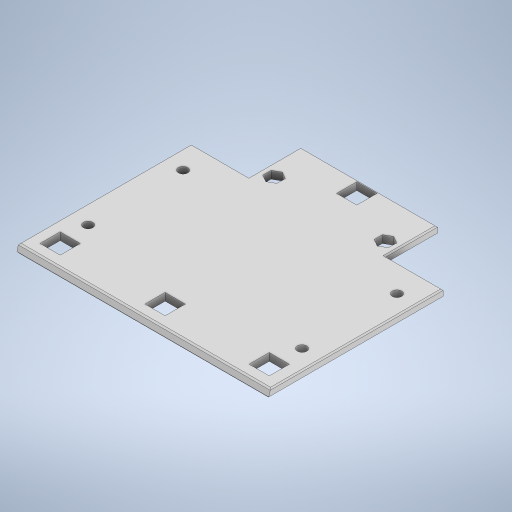
# Autodesk Inventor part: Plech pro celý spodek
Saved by Autodesk Inventor 2024 (Build 280153000, 153)
## iProperties
Created: 2023-09-06
Part Number: Plech pro celý spodek
Material: Všeobecné
Document SubType Name: Modeling
Designer: Simak
Density: 1 g/cm^3
Appearance: Výchozí
Author: Simak
Autodesk Inventor part; units mm, degrees
ref_plane "YZ Plane" through (0, 0, 0) normal (1, 0, 0) x (0, 1, 0)
ref_plane "XZ Plane" through (0, 0, 0) normal (0, 1, 0) x (-1, 0, 0)
ref_plane "XY Plane" through (0, 0, 0) normal (0, 0, 1) x (1, 0, 0)
sketch "Náčrt1" plane through (0, 0, 0) normal (0, 1, 0) x (-1, 0, 0)
  line L0 (49.75, -19.25) -> (49.75, 49.75)
  line L1 (49.75, 49.75) -> (-49.75, 49.75)
  line L2 (-49.75, 49.75) -> (-49.75, -19.25)
  line L3 (-49.75, -19.25) -> (-27, -19.25)
  line L4 (-27, -19.25) -> (-27, -49.75)
  line L5 (-27, -49.75) -> (27, -49.75)
  line L6 (27, -49.75) -> (27, -19.25)
  line L7 (27, -19.25) -> (49.75, -19.25)
  point P0 (0, 0)
  dimension "d0" = 30.5
  dimension "d1" = 99.5
  dimension "d2" = 22.75
  dimension "d3" = 99.5
  dimension "d4" = 54
  dimension "d5" = 49.75
  dimension "d6" = 49.75
  constraints: 16 end point, 6 perpendicular, 2 vertical, 1 parallel
  measures "d0" distance of L3.end L4.end
  measures "d1" distance of L0.end L1.end
  measures "d2" distance of L2.end L3.end
  measures "d3" distance between parallel lines of L1 L5
  measures "d4" distance of L4.end L5.end
  measures "d5" horizontal distance of L1.end point (0, 0)
  measures "d6" distance from line of point (0, 0) L1
extrude "Vysunutí1" add sketch "Náčrt1" along normal blind 3
sketch "Náčrt2" plane through (27, 0, -19.25) normal (1, 0, 0) x (0, 0, -1)
  line L0 (30.5, 3) -> (0, 3) projected
  line L1 (0, 3) -> (0, 11)
  line L2 (0, 11) -> (9.875, 11)
  line L3 (9.875, 11) -> (9.875, 7.646)
  arc A0 (9.875, 7.646) -> (20.625, 7.646) centre (15.25, 10.5828) ccw
  line L4 (20.625, 7.646) -> (20.625, 11)
  line L5 (20.625, 11) -> (30.5, 11)
  line L6 (30.5, 11) -> (30.5, 3)
  line L7 (0, 0) -> (30.5, 0) projected
  point P0 (-19.25, 0)
  dimension "d9" = 6.125
  dimension "d10" = 11
  dimension "d11" = 9.875
  dimension "d12" = 3.354
  constraints: 12 end point, 3 perpendicular, 2 equal length, 2 point on circle, 2 point on line, 1 centre point, 1 parallel, 1 vertical
  measures "d9" radius of A0
  measures "d10" distance between parallel lines of L5 L7
  measures "d11" distance of L4.end L5.end
  measures "d12" distance of L4.start L4.end
extrude "Vysunutí2" add sketch "Náčrt2" against normal up to surface (54 mm away)
sketch "Náčrt3" plane through (27, 3, -19.25) normal (0, 0, 1) x (1, 0, 0)
  line L0 (0, 8) -> (-54, 8) projected
  line L1 (-39, 8) -> (-39, 0)
  line L2 (-15, 8) -> (-15, 0)
  line L3 (-76.75, 0) -> (22.75, 0) projected
  line L4 (0, 8) -> (0, 0) projected
  line L5 (-54, 8) -> (-54, 0) projected
  line L6 (-15, 4) -> (0, 4)
  line L7 (-39, 4) -> (-54, 4)
  point P0 (-27, -3)
  dimension "d24" = 24
  constraints: 8 end point, 4 midpoint, 4 point on line, 2 vertical, 1 collinear
  measures "d24" distance between parallel lines of L1 L2
extrude "Vysunutí3" cut sketch "Náčrt3" against normal up to surface (20.625 mm away) contours L2 L3 L1 L0
sketch "Náčrt4" plane through (-27, 3, -19.25) normal (0, 0, 1) x (1, 0, 0)
  line L0 (0, 1.4578) -> (15, 1.4578) projected
  line L1 (39, 1.4578) -> (54, 1.4578) projected
  line L2 (10, 1.4578) -> (10, 8)
  line L3 (54, 8) -> (0, 8) projected
  line L4 (0, 8) -> (0, 0) projected
  line L5 (44, 8) -> (44, 1.4578)
  line L6 (54, 8) -> (54, 0) projected
  line L7 (15, 0) -> (15, 8) projected
  line L8 (39, 8) -> (39, 0) projected
  point P0 (27, -3)
  dimension "d20" = 10
  dimension "d21" = 10
  constraints: 4 end point, 4 point on line, 2 vertical
  measures "d20" distance between parallel lines of L4 L2
  measures "d21" distance between parallel lines of L6 L5
extrude "Vysunutí4" cut sketch "Náčrt4" against normal up to next contours L2 L3 L7 L0 | L8 L3 L5 L1
sketch "Náčrt5" plane through (-27, 3, -19.25) normal (0, 0, 1) x (1, 0, 0)
  line L0 (10, 1.4578) -> (10, 0)
  line L1 (15, 0) -> (0, 0) projected
  line L2 (44, 1.4578) -> (44, 0)
  line L3 (54, 0) -> (39, 0) projected
  line L4 (15, 1.4578) -> (10, 1.4578) projected
  line L5 (15, 0) -> (15, 1.4578) projected
  line L6 (-22.75, 0) -> (76.75, 0) projected
  line L7 (39, 1.4578) -> (39, 0) projected
  line L8 (44, 1.4578) -> (39, 1.4578) projected
  point P0 (27, -3)
  constraints: 4 end point, 2 coincident, 2 point on line, 1 parallel, 1 vertical
extrude "Vysunutí5" cut sketch "Náčrt5" against normal blind 6.875
sketch "Náčrt6" plane through (27, 7.646, -39.875) normal (0, 0, 1) x (1, 0, 0)
  line L0 (0, 3.354) -> (-54, 3.354) projected
  line L1 (-37, 3.354) -> (-37, -3.646)
  line L2 (-37, -3.646) -> (-17, -3.646)
  line L3 (-17, -3.646) -> (-17, 3.354)
  line L4 (-76.75, -4.646) -> (22.75, -4.646) projected
  line L5 (0, 3.354) -> (0, 0) projected
  line L6 (-17, -0.146) -> (0, -0.146) construction
  line L7 (-37, -0.146) -> (-54, -0.146) construction
  line L8 (-54, -7.646) -> (-54, 3.354) projected
  point P0 (-27, -7.646)
  dimension "d27" = 1
  dimension "d35" = 20
  constraints: 10 end point, 4 point on line, 2 horizontal, 2 midpoint, 2 perpendicular, 1 collinear, 1 vertical
  measures "d27" distance between parallel lines of L4 L2
  measures "d35" distance of L1.end L2.end
extrude "Vysunutí6" cut sketch "Náčrt6" against normal up to next
sketch "Náčrt7" plane through (-27, 11, -19.25) normal (0, 1, 0) x (1, 0, 0)
  circle A0 centre (5, 4.9375) radius 1.85
  circle A1 centre (5, 25.5625) radius 1.85
  circle A2 centre (49, 25.5625) radius 1.85
  circle A3 centre (49, 4.9375) radius 1.85
  line L0 (76.75, 0) -> (54, 0) projected
  line L1 (49, 4.9375) -> (54, 0) construction
  line L2 (54, 0) -> (44, 0) projected
  line L3 (44, 0) -> (49, 4.9375) construction
  line L4 (54, 9.875) -> (49, 4.9375) construction
  line L5 (10, 0) -> (10, 6.875) projected
  line L6 (5, 4.9375) -> (10, 0) construction
  line L7 (0, 30.5) -> (0, 0) projected
  line L8 (0, 0) -> (5, 4.9375) construction
  line L9 (5, 4.9375) -> (0, 9.875) construction
  line L10 (0, 20.625) -> (5, 25.5625) construction
  line L11 (5, 25.5625) -> (0, 30.5) construction
  line L12 (54, 0) -> (54, 30.5) projected
  line L13 (54, 20.625) -> (49, 25.5625) construction
  line L14 (49, 25.5625) -> (54, 30.5) construction
  point P0 (27, -19.25)
  dimension "d6" = 49.75
  dimension "d36" = 3.7
  constraints: 20 end point, 12 equal length, 4 centre point, 3 equal radius, 1 coincident
  measures "d36" diameter of A1
extrude "Vysunutí7" cut sketch "Náčrt7" against normal through all
sketch "Náčrt27" plane through (0, 0, 0) normal (0, -1, 0) x (1, 0, 0)
  circle A0 centre (22, -44.8125) radius 1.85 projected
  line L0 (19.175, -43.1815) -> (22, -41.5505)
  line L1 (22, -41.5505) -> (24.825, -43.1815)
  line L2 (24.825, -43.1815) -> (24.825, -46.4435)
  line L3 (24.825, -46.4435) -> (22, -48.0745)
  line L4 (22, -48.0745) -> (19.175, -46.4435)
  line L5 (19.175, -46.4435) -> (19.175, -43.1815)
  line L6 (19.175, -25.8185) -> (19.175, -22.5565)
  line L7 (19.175, -22.5565) -> (22, -20.9255)
  line L8 (22, -20.9255) -> (24.825, -22.5565)
  line L9 (24.825, -22.5565) -> (24.825, -25.8185)
  line L10 (24.825, -25.8185) -> (22, -27.4495)
  line L11 (22, -27.4495) -> (19.175, -25.8185)
  circle A1 centre (-22, -24.1875) radius 1.85 projected
  line L12 (-19.175, -25.8185) -> (-22, -27.4495)
  line L13 (-22, -27.4495) -> (-24.825, -25.8185)
  line L14 (-24.825, -25.8185) -> (-24.825, -22.5565)
  line L15 (-24.825, -22.5565) -> (-22, -20.9255)
  line L16 (-22, -20.9255) -> (-19.175, -22.5565)
  line L17 (-19.175, -22.5565) -> (-19.175, -25.8185)
  circle A2 centre (-22, -44.8125) radius 1.85 projected
  line L18 (-19.175, -46.4435) -> (-22, -48.0745)
  line L19 (-22, -48.0745) -> (-24.825, -46.4435)
  line L20 (-24.825, -46.4435) -> (-24.825, -43.1815)
  line L21 (-24.825, -43.1815) -> (-22, -41.5505)
  line L22 (-22, -41.5505) -> (-19.175, -43.1815)
  line L23 (-19.175, -43.1815) -> (-19.175, -46.4435)
  point P0 (0, 0)
  point P1 (22, -24.1875)
  dimension "d179" = 5.65
  constraints: 48 end point, 4 vertical, 3 coincident, 3 equal length, 1 horizontal alignment, 1 vertical alignment, 52 other
  measures "d179" distance between parallel lines of L2 L5
extrude "Vysunutí30" cut sketch "Náčrt27" against normal blind 7 contours A0 | L0 L1 L2 L3 L4 L5 | L6 L7 L8 L9 L10 L11 | A1 | L12 L13 L14 L15 L16 L17 | A2 | L18 L19 L20 L21 L22 L23
chamfer "Zkosení2" distance 1 angle 45 4 edges at (20.15, 7, -44.8125) (20.15, 7, -24.1875) (-23.85, 7, -24.1875) (-23.85, 7, -44.8125)
sketch "Náčrt28" plane through (0, 3, 0) normal (0, 1, 0) x (1, 0, 0)
  circle A0 centre (-42.25, 8.5) radius 1.85
  circle A1 centre (42.25, 8.5) radius 1.85
  circle A2 centre (42.25, -29) radius 1.85
  circle A3 centre (-42.25, -29) radius 1.85
  line L0 (-42.25, 8.5) -> (-49.75, 8.5) construction
  line L1 (-49.75, 19.25) -> (-49.75, -49.75) projected
  line L2 (42.25, 8.5) -> (49.75, 8.5) construction
  line L3 (49.75, -49.75) -> (49.75, 19.25) projected
  line L4 (-49.75, -49.75) -> (49.75, -49.75) projected
  point P0 (0, 0)
  dimension "d185" = 3.7
  dimension "d186" = 84.5
  dimension "d187" = 37.5
  dimension "d195" = 20.75
  constraints: 4 centre point, 4 end point, 3 equal radius, 3 point on line, 2 horizontal alignment, 2 vertical alignment, 1 collinear, 1 horizontal
  measures "d185" diameter of A0
  measures "d186" distance of L2.start L0.start
  measures "d187" distance of A3.centre L0.start
  measures "d195" distance from line of L4 A3.centre
sketch "Náčrt29" plane through (49.75, 0, 49.75) normal (1, 0, 0) x (0, 0, -1)
  line L0 (0, 0) -> (69, 0) projected
  line L1 (0, 0) -> (6.6987, 25)
  line L2 (6.6987, 25) -> (9.8046, 25)
  line L3 (9.8046, 25) -> (3.9097, 3)
  line L4 (0, 3) -> (69, 3) projected
  line L5 (0, 0) -> (0, 3) projected
  point P0 (49.75, 0)
  point P1 (0.8038, 3)
  dimension "d188" = 75
  dimension "d189" = 25
  dimension "d190" = 3
  constraints: 6 end point, 1 horizontal, 1 parallel, 1 point on line
  measures "d188" angle of L0 L1
  measures "d189" distance between parallel lines of L0 L2
  measures "d190" distance between parallel lines of L1 L3
extrude "Vysunutí31" add sketch "Náčrt29" against normal up to surface (99.5 mm away) contours L1 L2 L3 L4
extrude "Vysunutí32" cut sketch "Náčrt29" against normal through all contours L5 L4 L1
extrude "Vysunutí33" cut sketch "Náčrt28" against normal up to next
sketch "Náčrt31" plane through (0, 3, 0) normal (0, 1, 0) x (1, 0, 0)
  line L0 (37.136, -36.833) -> (45.136, -36.833)
  line L1 (45.136, -36.833) -> (45.136, -44.833)
  line L2 (45.136, -44.833) -> (37.136, -44.833)
  line L3 (37.136, -44.833) -> (37.136, -36.833)
  line L4 (-4, -36.833) -> (4, -36.833)
  line L5 (4, -36.833) -> (4, -44.833)
  line L6 (4, -44.833) -> (-4, -44.833)
  line L7 (-4, -44.833) -> (-4, -36.833)
  line L8 (-45.463, -36.833) -> (-37.463, -36.833)
  line L9 (-37.463, -36.833) -> (-37.463, -44.833)
  line L10 (-37.463, -44.833) -> (-45.463, -44.833)
  line L11 (-45.463, -44.833) -> (-45.463, -36.833)
  line L12 (49.75, -45.8403) -> (49.75, 19.25) projected
  line L13 (-49.75, 19.25) -> (-49.75, -45.8403) projected
  line L14 (-49.75, -49.75) -> (49.75, -49.75) projected
  line L15 (4, 38.875) -> (-4, 38.875)
  line L16 (-4, 38.875) -> (-4, 30.875)
  line L17 (-4, 30.875) -> (4, 30.875)
  line L18 (4, 30.875) -> (4, 38.875)
  line L19 (27, 39.875) -> (10, 39.875) projected
  line L20 (4, 34.875) -> (27, 34.875) construction
  line L21 (-4, 34.875) -> (-27, 34.875) construction
  line L22 (-27, 49.75) -> (-27, 19.25) projected
  line L23 (27, 19.25) -> (27, 49.75) projected
  point P0 (0, 0)
  point P1 (0, -36.833)
  dimension "d198" = 8
  dimension "d199" = 4.614
  dimension "d200" = 4.287
  dimension "d201" = 4.917
  dimension "d334" = 1
  constraints: 36 end point, 8 equal length, 8 parallel, 6 horizontal, 4 perpendicular, 3 midpoint, 3 point on line, 2 horizontal alignment, 1 vertical alignment
  measures "d198" distance between parallel lines of L2 L0
  measures "d199" distance between parallel lines of L12 L1
  measures "d200" distance between parallel lines of L13 L11
  measures "d201" distance from line of L14 L5.end
  measures "d334" distance between parallel lines of L15 L19
extrude "Vysunutí34" cut sketch "Náčrt31" against normal up to next
sketch "Náčrt32" plane through (-27, 0, -19.25) normal (0, 0, -1) x (-1, 0, 0)
  line L0 (0, 0) -> (22.75, 0) projected
  line L1 (22.75, 0) -> (20.25, 0)
  line L2 (20.25, 0) -> (20.25, 25)
  line L3 (20.25, 25) -> (22.75, 25)
  line L4 (22.75, 25) -> (22.75, 0)
  line L5 (-76.75, 0) -> (-74.25, 0)
  line L6 (-74.25, 0) -> (-74.25, 25)
  line L7 (-74.25, 25) -> (-76.75, 25)
  line L8 (-76.75, 25) -> (-76.75, 0)
  line L9 (-76.75, 25) -> (22.75, 25) projected
  point P0 (-27, 0)
  point P1 (20.25, 0)
  dimension "d204" = 2.5
  constraints: 16 end point, 4 parallel, 2 horizontal, 2 perpendicular, 1 collinear, 1 point on line
  measures "d204" distance between parallel lines of L2 L4
extrude "Vysunutí35" add sketch "Náčrt32" against normal up to next
sketch "Náčrt34" plane through (0, 3, 0) normal (0, 1, 0) x (1, 0, 0)
  circle A0 centre (42.25, -29) radius 1.85 projected
  circle A1 centre (42.25, 8.5) radius 1.85 projected
  circle A2 centre (-42.25, 8.5) radius 1.85 projected
  circle A3 centre (-42.25, -29) radius 1.85 projected
  circle A4 centre (42.25, -29) radius 3.5
  circle A5 centre (42.25, 8.5) radius 3.5
  circle A6 centre (-42.25, 8.5) radius 3.5
  circle A7 centre (-42.25, -29) radius 3.5
  point P0 (0, 0)
  dimension "d214" = 7
  constraints: 4 centre point, 4 coincident, 3 equal radius
  measures "d214" diameter of A4
extrude "Vysunutí37" add sketch "Náčrt34" along normal blind 4
sketch "Náčrt35" plane through (0, 0, 0) normal (0, -1, 0) x (1, 0, 0)
  line L0 (19.175, -25.8185) -> (19.175, -22.5565) projected
  circle A0 centre (42.25, -8.5) radius 1.85 projected
  line L1 (39.425, -10.131) -> (39.425, -6.869)
  line L2 (39.425, -6.869) -> (42.25, -5.238)
  line L3 (42.25, -5.238) -> (45.075, -6.869)
  line L4 (45.075, -6.869) -> (45.075, -10.131)
  line L5 (45.075, -10.131) -> (42.25, -11.762)
  line L6 (42.25, -11.762) -> (39.425, -10.131)
  circle A1 centre (42.25, 29) radius 1.85 projected
  line L7 (39.425, 27.369) -> (39.425, 30.631)
  line L8 (39.425, 30.631) -> (42.25, 32.262)
  line L9 (42.25, 32.262) -> (45.075, 30.631)
  line L10 (45.075, 30.631) -> (45.075, 27.369)
  line L11 (45.075, 27.369) -> (42.25, 25.738)
  line L12 (42.25, 25.738) -> (39.425, 27.369)
  circle A2 centre (-42.25, 29) radius 1.85 projected
  line L13 (-45.075, 27.369) -> (-45.075, 30.631)
  line L14 (-45.075, 30.631) -> (-42.25, 32.262)
  line L15 (-42.25, 32.262) -> (-39.425, 30.631)
  line L16 (-39.425, 30.631) -> (-39.425, 27.369)
  line L17 (-39.425, 27.369) -> (-42.25, 25.738)
  line L18 (-42.25, 25.738) -> (-45.075, 27.369)
  circle A3 centre (-42.25, -8.5) radius 1.85 projected
  line L19 (-45.075, -10.131) -> (-45.075, -6.869)
  line L20 (-45.075, -6.869) -> (-42.25, -5.238)
  line L21 (-42.25, -5.238) -> (-39.425, -6.869)
  line L22 (-39.425, -6.869) -> (-39.425, -10.131)
  line L23 (-39.425, -10.131) -> (-42.25, -11.762)
  line L24 (-42.25, -11.762) -> (-45.075, -10.131)
  point P0 (0, 0)
  constraints: 48 end point, 4 coincident, 4 equal length, 4 vertical, 52 other
extrude "Vysunutí38" [suppressed]
chamfer "Zkosení3" [suppressed]
sketch "Náčrt36" plane through (42.25, 7, -8.5) normal (0, 1, 0) x (1, 0, 0)
  circle A0 centre (0, 0) radius 3.5 projected
  line L0 (0, -3.5) -> (5, -3.5)
  line L1 (5, -54.3403) -> (5, 10.75) projected
  line L2 (0, 3.5) -> (5, 3.5)
  line L3 (0, -34) -> (5, -34)
  circle A1 centre (0, -37.5) radius 3.5 projected
  line L4 (0, -41) -> (5, -41)
  line L5 (-84.5, -41) -> (-89.5, -41)
  line L6 (-89.5, 10.75) -> (-89.5, -54.3403) projected
  circle A2 centre (-84.5, -37.5) radius 3.5 projected
  line L7 (-84.5, -34) -> (-89.5, -34)
  circle A3 centre (-84.5, 0) radius 3.5 projected
  line L8 (-84.5, -3.5) -> (-89.5, -3.5)
  line L9 (-84.5, 3.5) -> (-89.5, 3.5)
  point P0 (-42.25, -8.5)
  point P1 (-84.5, 3.5)
  point P2 (5, 3.5)
  point P3 (0, 3.5)
  dimension "d6" = 49.75
  constraints: 16 end point, 8 horizontal, 6 point on line, 4 perpendicular, 4 tangent, 3 parallel, 3 vertical alignment, 2 point on circle, 4 other
extrude "Vysunutí39" add sketch "Náčrt36" against normal up to next contours A0 L2 L1 L0 | L4 A1 L3 L1 | L5 L6 L7 A2 | L9 A3 L8 L6
sketch "Náčrt37" plane through (27, 7.646, -39.875) normal (0, 0, 1) x (1, 0, 0)
  line L0 (-15, -4.646) -> (-39, -4.646) projected
  line L1 (-15, 0) -> (-15, -4.646) projected
  line L2 (-39, -4.646) -> (-39, 0) projected
  line L3 (-39, 0) -> (-39, 3.354)
  line L4 (-37, 3.354) -> (-54, 3.354) projected
  line L5 (-15, 0) -> (-15, 3.354)
  line L6 (-15, 3.354) -> (-17.0063, 3.354)
  line L7 (-17.0063, 3.354) -> (-37, 3.354)
  point P0 (-27, -7.646)
  constraints: 8 end point, 2 vertical, 1 collinear, 1 perpendicular, 1 point on line
extrude "Vysunutí40" cut sketch "Náčrt37" against normal up to next
sketch "Náčrt40" plane through (47.25, 3, -19.25) normal (-1, 0, 0) x (0, 0, 1)
  line L0 (0, -3) -> (0, 22) projected
  line L1 (0, 0) -> (1, 0)
  line L2 (1, 0) -> (1, 10)
  line L3 (1, 10) -> (0, 10)
  line L4 (0, 10) -> (0, 0)
  line L5 (0, 0) -> (7.25, 0) projected
  point P0 (19.25, -3)
  point P1 (0, 10)
  dimension "d236" = 1
  dimension "d237" = 10
  constraints: 8 end point, 2 parallel, 1 horizontal, 1 perpendicular
  measures "d236" distance of L2.end L3.end
  measures "d237" distance between parallel lines of L5 L3
extrude "Vysunutí41" add sketch "Náčrt40" along normal blind 22
sketch "Náčrt41" plane through (-47.25, 3, -19.25) normal (1, 0, 0) x (0, 0, -1)
  line L0 (-1, 10) -> (0, 10) projected
  line L1 (0, 10) -> (0, 8) projected
  line L2 (0, 0) -> (0, 8) projected
  line L3 (-1, 0) -> (0, 0) projected
  line L4 (-1, 0) -> (-1, 10) projected
  point P0 (-19.25, -3)
extrude "Vysunutí42" add sketch "Náčrt41" along normal blind 22
sketch "Náčrt42" plane through (0, 3, 0) normal (0, 1, 0) x (1, 0, 0)
  line L0 (-25.25, 18.25) -> (-47.25, 18.25) projected
  line L1 (-47.25, 18.25) -> (-47.25, 12) projected
  line L2 (-47.25, 12) -> (-42.25, 12) projected
  arc A0 (-42.25, 5) -> (-42.25, 12) centre (-42.25, 8.5) ccw projected
  line L3 (-42.25, 5) -> (-47.25, 5) projected
  line L4 (-47.25, 5) -> (-47.25, -25.5) projected
  line L5 (-47.25, -25.5) -> (-42.25, -25.5) projected
  arc A1 (-42.25, -32.5) -> (-42.25, -25.5) centre (-42.25, -29) ccw projected
  line L6 (-42.25, -32.5) -> (-47.25, -32.5) projected
  line L7 (-47.25, -32.5) -> (-47.25, -45.8403) projected
  line L8 (-47.25, -45.8403) -> (47.25, -45.8403) projected
  line L9 (47.25, -45.8403) -> (47.25, -32.5) projected
  line L10 (47.25, -32.5) -> (42.25, -32.5) projected
  arc A2 (42.25, -25.5) -> (42.25, -32.5) centre (42.25, -29) ccw projected
  line L11 (42.25, -25.5) -> (47.25, -25.5) projected
  line L12 (47.25, -25.5) -> (47.25, 5) projected
  line L13 (47.25, 5) -> (42.25, 5) projected
  arc A3 (42.25, 12) -> (42.25, 5) centre (42.25, 8.5) ccw projected
  line L14 (42.25, 12) -> (47.25, 12) projected
  line L15 (47.25, 12) -> (47.25, 18.25) projected
  line L16 (47.25, 18.25) -> (25.25, 18.25) projected
  line L17 (25.25, 18.25) -> (25.25, 19.25) projected
  line L18 (25.25, 19.25) -> (17, 19.25) projected
  line L19 (17, 19.25) -> (17, 26.125) projected
  line L20 (17, 26.125) -> (12, 26.125) projected
  line L21 (12, 26.125) -> (12, 49.75) projected
  line L22 (-12, 49.75) -> (12, 49.75) projected
  line L23 (-12, 26.125) -> (-12, 49.75) projected
  line L24 (-12, 26.125) -> (-17, 26.125) projected
  line L25 (-17, 19.25) -> (-17, 26.125) projected
  line L26 (-17, 19.25) -> (-25.25, 19.25) projected
  line L27 (-25.25, 19.25) -> (-25.25, 18.25) projected
  line L28 (-37.463, -36.833) -> (-37.463, -44.833) projected
  line L29 (-37.463, -44.833) -> (-45.463, -44.833) projected
  line L30 (-45.463, -44.833) -> (-45.463, -36.833) projected
  line L31 (-45.463, -36.833) -> (-37.463, -36.833) projected
  line L32 (4, -36.833) -> (4, -44.833) projected
  line L33 (4, -44.833) -> (-4, -44.833) projected
  line L34 (-4, -44.833) -> (-4, -36.833) projected
  line L35 (-4, -36.833) -> (4, -36.833) projected
  line L36 (45.136, -36.833) -> (45.136, -44.833) projected
  line L37 (45.136, -44.833) -> (37.136, -44.833) projected
  line L38 (37.136, -44.833) -> (37.136, -36.833) projected
  line L39 (37.136, -36.833) -> (45.136, -36.833) projected
  line L40 (12, 34.5) -> (17, 34.5) projected
  line L41 (-17, 34.5) -> (-12, 34.5) projected
  line L42 (45.75, 3.5) -> (45.75, -24)
  line L43 (45.75, -24) -> (42.25, -24)
  arc A4 (42.25, -24) -> (42.25, -34) centre (42.25, -29) ccw
  line L44 (42.25, -34) -> (45.75, -34)
  line L45 (45.75, -34) -> (45.75, -44.3403)
  line L46 (45.75, -44.3403) -> (-45.75, -44.3403)
  line L47 (-45.75, -44.3403) -> (-45.75, -34)
  line L48 (-45.75, -34) -> (-42.25, -34)
  arc A5 (-42.25, -34) -> (-42.25, -24) centre (-42.25, -29) ccw
  line L49 (-42.25, -24) -> (-45.75, -24)
  line L50 (-45.75, -24) -> (-45.75, 3.5)
  line L51 (-45.75, 3.5) -> (-42.25, 3.5)
  arc A6 (-42.25, 3.5) -> (-42.25, 13.5) centre (-42.25, 8.5) ccw
  line L52 (-42.25, 13.5) -> (-45.75, 13.5)
  line L53 (-45.75, 13.5) -> (-45.75, 16.75)
  line L54 (-45.75, 16.75) -> (-23.75, 16.75)
  line L55 (-23.75, 16.75) -> (-23.75, 17.75)
  line L56 (-23.75, 17.75) -> (-15.5, 17.75)
  line L57 (-15.5, 17.75) -> (-15.5, 24.625)
  line L58 (-15.5, 24.625) -> (-10.5, 24.625)
  line L59 (-10.5, 24.625) -> (-10.5, 48.25)
  line L60 (-10.5, 48.25) -> (10.5, 48.25)
  line L61 (10.5, 48.25) -> (10.5, 24.625)
  line L62 (10.5, 24.625) -> (15.5, 24.625)
  line L63 (15.5, 24.625) -> (15.5, 17.75)
  line L64 (15.5, 17.75) -> (23.75, 17.75)
  line L65 (23.75, 17.75) -> (23.75, 16.75)
  line L66 (23.75, 16.75) -> (45.75, 16.75)
  line L67 (45.75, 16.75) -> (45.75, 13.5)
  line L68 (45.75, 13.5) -> (42.25, 13.5)
  arc A7 (42.25, 13.5) -> (42.25, 3.5) centre (42.25, 8.5) ccw
  line L69 (42.25, 3.5) -> (45.75, 3.5)
  line L70 (36.136, -35.833) -> (36.136, -45.833)
  line L71 (36.136, -45.833) -> (46.136, -45.833)
  line L72 (46.136, -45.833) -> (46.136, -35.833)
  line L73 (46.136, -35.833) -> (36.136, -35.833)
  line L74 (5, -35.833) -> (5, -45.833)
  line L75 (5, -45.833) -> (-5, -45.833)
  line L76 (-5, -45.833) -> (-5, -35.833)
  line L77 (-5, -35.833) -> (5, -35.833)
  line L78 (-36.463, -45.833) -> (-36.463, -35.833)
  line L79 (-36.463, -35.833) -> (-46.463, -35.833)
  line L80 (-46.463, -35.833) -> (-46.463, -45.833)
  line L81 (-46.463, -45.833) -> (-36.463, -45.833)
  line L82 (-42.25, -34) -> (-42.25, -35.833)
  line L83 (42.25, -34) -> (42.25, -35.833)
  line L84 (42.25, 13.5) -> (42.25, 16.75)
  line L85 (-42.25, 13.5) -> (-42.25, 16.75)
  line L86 (4, 30.875) -> (-4, 30.875) projected
  line L87 (4, 38.875) -> (4, 30.875) projected
  line L88 (-4, 30.875) -> (-4, 38.875) projected
  line L89 (-5, 39.875) -> (-5, 29.875)
  line L90 (-5, 29.875) -> (5, 29.875)
  line L91 (5, 29.875) -> (5, 39.875)
  line L92 (27, 39.875) -> (12, 39.875) projected
  line L93 (12, 39.875) -> (-12, 39.875)
  line L94 (12, 38.375) -> (-12, 38.375)
  line L95 (12, 39.875) -> (12, 34.5) projected
  line L96 (-12, 34.5) -> (-12, 39.875) projected
  point P0 (0, 0)
  point P1 (-36.463, -44.3403)
  point P2 (-5, -44.3403)
  point P3 (5, -44.3403)
  point P4 (36.136, -44.3403)
  point P5 (-45.75, -35.833)
  point P6 (45.75, -35.833)
  point P7 (4, 38.375)
  point P8 (-4, 38.375)
  point P9 (10.5, 38.375)
  point P10 (5, 38.375)
  point P11 (-5, 38.375)
  point P12 (-10.5, 38.375)
  point P13 (4, -44.3403)
  point P14 (-4, -44.3403)
  dimension "d242" = 1.5
  dimension "d243" = 1
  dimension "d244" = 1
  dimension "d245" = 1
  dimension "d336" = 1
  dimension "d337" = 1.5
  constraints: 98 end point, 11 point on line, 8 point on circle, 4 centre point, 3 perpendicular, 1 parallel, 42 other
  measures "d242" distance between parallel lines of L12 L42
  measures "d243" distance between parallel lines of L38 L70
  measures "d244" distance between parallel lines of L35 L77
  measures "d245" distance between parallel lines of L28 L78
  measures "d336" distance between parallel lines of L86 L90
  measures "d337" distance between parallel lines of L93 L94
extrude "Vysunutí43" [suppressed]
sketch "Náčrt44" plane through (-49.75, 25, 43.0513) normal (0, 1, 0) x (1, 0, 0)
  line L0 (97, 3.1058) -> (2.5, 3.1058) projected
  line L1 (32.781, 3.1058) -> (32.781, 11.1058)
  line L2 (24.781, 11.1058) -> (24.781, 3.1058)
  line L3 (0, 62.3013) -> (0, 0) projected
  line L4 (32.781, 11.1058) -> (24.781, 11.1058)
  point P0 (49.75, 43.0513)
  point P1 (0, 18.7254)
  point P2 (28.781, 11.1058)
  dimension "d266" = 8
  dimension "d267" = 28.781
  constraints: 6 end point, 2 perpendicular, 2 point on line, 1 horizontal, 1 midpoint, 1 vertical
  measures "d266" distance between parallel lines of L0 L4
  measures "d267" distance from line of point (28.781, 11.106) L3
extrude "Vysunutí45" add sketch "Náčrt44" against normal blind 6
sketch "Náčrt46" plane through (-24.969, 25, 31.9454) normal (-1, 0, 0) x (0, 0, 1)
  line L0 (0, -6) -> (8, -6) projected
  line L1 (8, -6) -> (9.6077, -6)
  line L2 (8, 0) -> (13.8949, -22) projected
  line L3 (8, 0) -> (8, -6) projected
  point P0 (-31.9454, -25)
  constraints: 2 end point, 1 horizontal, 1 point on line
extrude "Vysunutí46" add sketch "Náčrt46" against normal up to surface (8 mm away)
chamfer "Zkosení8" distance 9.6 angle 45 1 edges at (-20.969, 19, 41.5531)
sketch "Náčrt45" plane through (-49.75, 25, 43.0513) normal (0, 1, 0) x (1, 0, 0)
  line L0 (32.781, 3.1058) -> (24.781, 3.1058) projected
  line L1 (24.781, 11.1058) -> (24.781, 3.1058) projected
  line L2 (32.781, 11.1058) -> (24.781, 11.1058) projected
  line L3 (99.5, 0) -> (0, 0) projected
  point P0 (49.75, 43.0513)
  point P1 (28.781, 6.196)
  point P2 (28.781, 11.1058)
  dimension "d283" = 6.196
  constraints: 1 midpoint, 1 vertical alignment
  measures "d283" distance from line of point (28.781, 6.196) L3
hole "Díra1" at (-20.969, 25, 36.8553) direction (0, -1, 0) diameter 3.5 end up to surface
sketch "Náčrt47" plane through (-16.969, 25, 31.9454) normal (0, 0, -1) x (-1, 0, 0)
  line L0 (1.2, -1.4) -> (6.8, -1.4)
  line L1 (6.8, -1.4) -> (6.8, -4.6)
  line L2 (6.8, -4.6) -> (1.2, -4.6)
  line L3 (1.2, -4.6) -> (1.2, -1.4)
  line L4 (0, 0) -> (8, 0) projected
  line L5 (0, 0) -> (0, -6) projected
  point P0 (-16.969, -25)
  point P1 (4, -1.4)
  point P2 (4, 0)
  point P3 (0, -3)
  point P4 (1.2, -3)
  dimension "d279" = 5.6
  dimension "d280" = 3.2
  constraints: 8 end point, 4 midpoint, 2 parallel, 1 horizontal, 1 horizontal alignment, 1 perpendicular, 1 vertical alignment
  measures "d279" distance of L1.end L2.end
  measures "d280" distance of L0.end L1.end
extrude "Vysunutí47" cut sketch "Náčrt47" against normal blind 8.5
sketch "Náčrt48" plane through (-49.75, 0, -19.25) normal (-1, 0, 0) x (0, 0, 1)
  line L0 (0, 25) -> (62.3013, 25) projected
  line L1 (0, 25) -> (24.25, 44)
  line L2 (24.25, 44) -> (24.25, 25)
  line L3 (0, 25) -> (62.3013, 25) projected
  point P0 (19.25, 0)
  dimension "d285" = 24.25
  dimension "d286" = 19
  constraints: 4 end point, 1 perpendicular, 1 point on line
  measures "d285" distance of L2.end L0.start
  measures "d286" distance of L1.end L2.end
extrude "Vysunutí48" add sketch "Náčrt48" against normal up to surface (2.5 mm away)
sketch "Náčrt49" plane through (-49.75, 25, 5) normal (0, 0, 1) x (1, 0, 0)
  line L0 (0, 0) -> (2.5, 0) projected
  line L1 (1.25, 0) -> (4.45, 0)
  line L2 (4.45, 0) -> (4.45, 5.2)
  line L3 (4.45, 5.2) -> (1.25, 5.2)
  line L4 (1.25, 5.2) -> (1.25, 0)
  line L5 (2.5, 7.2) -> (6.45, 7.2)
  line L6 (6.45, 7.2) -> (6.45, -2)
  line L7 (6.45, -2) -> (2.5, -2)
  line L8 (2.5, 7.2) -> (2.5, 5.2)
  line L9 (2.5, 0) -> (2.5, -12) projected
  line L10 (2.5, 0) -> (2.5, -2)
  line L11 (2.5, 0) -> (2.5, 19) projected
  point P0 (49.75, -25)
  point P1 (1.25, 0)
  point P2 (2.5, 0)
  point P3 (2.5, 0)
  dimension "d289" = 3.2
  dimension "d290" = 5.2
  dimension "d291" = 2
  dimension "d292" = 2
  dimension "d293" = 2
  constraints: 18 end point, 3 perpendicular, 2 collinear, 2 horizontal, 2 midpoint, 2 parallel, 1 point on line, 1 vertical, 1 vertical alignment
  measures "d289" distance of L2.end L3.end
  measures "d290" distance of L1.end L2.end
  measures "d291" distance between parallel lines of L1 L7
  measures "d292" distance between parallel lines of L6 L2
  measures "d293" distance between parallel lines of L3 L5
extrude "Vysunutí49" add sketch "Náčrt49" against normal blind 12.2
extrude "Vysunutí50" cut sketch "Náčrt49" against normal blind 10.2 contours L4 L3 L11 L0 | L11 L3 L2 L1
chamfer "Zkosení5" distance 1.8 angle 45 1 edges at (-45.3, 30.2, -0.1)
chamfer "Zkosení6" distance 3.95 angle 45 1 edges at (-47.25, 23, -1.1)
chamfer "Zkosení7" distance 2 angle 45 3 edges at (-43.3, 32.2, -1.1) (-43.3, 23, -7.2) (-43.3, 27.6, -7.2)
mirror "Zrcadlit1" about plane through (0, 0, 0) normal (1, 0, 0) of "Vysunutí45", "Vysunutí46", "Zkosení8", "Díra1", "Vysunutí47", "Vysunutí48", "Vysunutí49", "Vysunutí50", "Zkosení5", "Zkosení7"
chamfer "Zkosení11" distance 3.95 angle 45 1 edges at (47.25, 23, -1.1)
sketch "Náčrt33" plane through (-49.75, 0, -19.25) normal (-1, 0, 0) x (0, 0, 1)
  line L0 (36.318, 10.36) -> (42.098, 10.36) construction
  line L1 (36.318, 8.78) -> (42.098, 8.78)
  line L2 (42.098, 11.94) -> (36.318, 11.94)
  arc A0 (36.318, 11.94) -> (36.318, 8.78) centre (36.318, 10.36) ccw
  arc A1 (42.098, 8.78) -> (42.098, 11.94) centre (42.098, 10.36) ccw
  line L3 (0, 0) -> (69, 0) projected
  line L4 (0, 0) -> (0, 25) projected
  line L5 (36.318, 14.44) -> (42.098, 14.44)
  arc A2 (42.098, 6.28) -> (42.098, 14.44) centre (42.098, 10.36) ccw
  line L6 (42.098, 6.28) -> (36.318, 6.28)
  arc A3 (36.318, 14.44) -> (36.318, 6.28) centre (36.318, 10.36) ccw
  point P0 (19.25, 0)
  point P1 (39.208, 10.36)
  point P2 (34.738, 10.36)
  point P3 (43.678, 10.36)
  dimension "d207" = 8.78
  dimension "d208" = 3.16
  dimension "d209" = 8.94
  dimension "d210" = 34.738
  dimension "d211" = 2.5
  constraints: 12 end point, 10 point on circle, 4 centre point, 4 tangent, 2 parallel, 1 horizontal, 1 midpoint, 3 other
  measures "d207" distance between parallel lines of L3 L1
  measures "d208" distance between parallel lines of L1 L2
  measures "d209" distance of point (34.738, 10.36) point (43.678, 10.36)
  measures "d210" distance from line of L4 point (34.738, 10.36)
  measures "d211" distance between parallel lines of L2 L5
extrude "Vysunutí36" cut sketch "Náčrt33" along normal mid plane 10 contours A0 L2 A1 L1 | L5 A2 L6 A3
sketch "Náčrt50" plane through (-27, 0, -49.75) normal (-1, 0, 0) x (0, 0, 1)
  line L0 (0, 0) -> (0, 11) projected
  line L1 (0, 0) -> (30.5, 0) projected
  line L2 (0, 11) -> (0, 3) projected
  line L3 (0, 5.5) -> (10, 0)
  line L4 (0, 6.5) -> (3, 3.85)
  point P0 (49.75, 0)
  point P1 (0, 5.5)
  point P2 (0, 6.5)
  dimension "d316" = 5.5
  dimension "d317" = 10
  dimension "d318" = 6.5
  dimension "d319" = 3
  constraints: 4 end point, 4 point on line
  measures "d316" distance of L0.start L3.start
  measures "d317" distance of L0.start L3.end
  measures "d318" distance of L0.start L4.start
  measures "d319" distance from line of L0 L4.end
extrude "Vysunutí51" cut sketch "Náčrt50" against normal through all
sketch "Náčrt51" plane through (12, 7.646, -39.875) normal (-1, 0, 0) x (0, 0, 1)
  line L0 (-9.875, 3.354) -> (0, 3.354) projected
  line L1 (-9.875, 3.354) -> (0, 3.354)
  line L2 (0, 3.354) -> (0, -4.646)
  line L3 (-9.875, -1.146) -> (-9.875, 3.354)
  line L4 (-6.875, -3.796) -> (-5.3295, -4.646) projected
  line L5 (-9.875, -1.146) -> (-6.875, -3.796) projected
  line L6 (13.75, -4.646) -> (-5.3295, -4.646) projected
  point P0 (39.875, -7.646)
  point P1 (-9.875, -1.146)
  constraints: 6 end point, 2 point on line, 1 coincident, 1 horizontal, 1 parallel, 1 perpendicular
extrude "Vysunutí52" add sketch "Náčrt51" along normal up to next
sketch "Náčrt52" plane through (27, 11, -39.875) normal (0, 1, 0) x (1, 0, 0)
  line L0 (-15, 0) -> (-39, 0) projected
  line L1 (0, 9.875) -> (-54, 9.875) projected
  line L2 (-21.75, 0) -> (-32.25, 0)
  line L3 (-32.25, 0) -> (-32.25, 9.875)
  line L4 (-32.25, 9.875) -> (-21.75, 9.875)
  line L5 (-21.75, 9.875) -> (-21.75, 0)
  line L6 (-32.25, 4.9375) -> (-54, 4.9375) construction
  line L7 (-54, 6.875) -> (-54, -0.125) projected
  line L8 (-21.75, 4.9375) -> (0, 4.9375) construction
  line L9 (0, 9.875) -> (0, 0) projected
  point P0 (-27, -39.875)
  point P1 (-21.75, 9.875)
  point P2 (-32.25, 0)
  dimension "d323" = 10.5
  constraints: 12 end point, 4 point on line, 3 midpoint, 2 horizontal, 2 parallel, 1 collinear, 1 perpendicular
  measures "d323" distance between parallel lines of L3 L5
extrude "Vysunutí53" add sketch "Náčrt52" along normal blind 1
sketch "Náčrt53" plane through (0, 0, 0) normal (0, -1, 0) x (1, 0, 0)
  line L0 (5.25, -49.75) -> (-5.25, -49.75) projected
  line L1 (-5.25, -49.75) -> (-5.25, -39.875) projected
  line L2 (-5.25, -39.875) -> (5.25, -39.875) projected
  line L3 (5.25, -39.875) -> (5.25, -49.75) projected
  line L4 (0, -48.0745) -> (-2.825, -46.4435)
  line L5 (-2.825, -46.4435) -> (-2.825, -43.1815)
  line L6 (-2.825, -43.1815) -> (0, -41.5505)
  line L7 (0, -41.5505) -> (2.825, -43.1815)
  line L8 (2.825, -43.1815) -> (2.825, -46.4435)
  line L9 (2.825, -46.4435) -> (0, -48.0745)
  line L10 (-19.175, -46.4435) -> (-19.175, -43.1815) projected
  line L11 (0, -48.0745) -> (0, -49.75) construction
  line L12 (0, -41.5505) -> (0, -39.875) construction
  circle A0 centre (0, -44.8125) radius 1.85
  point P0 (0, 0)
  point P1 (0, -44.8125)
  dimension "d328" = 3.7
  constraints: 16 end point, 2 equal length, 2 midpoint, 1 centre point, 1 coincident, 1 vertical, 1 vertical alignment, 13 other
  measures "d328" diameter of A0
extrude "Vysunutí54" cut sketch "Náčrt53" against normal blind 10 contours L4 L5 L6 L7 L8 L9 | A0
extrude "Vysunutí55" cut sketch "Náčrt53" against normal up to next contours A0
sketch "Náčrt54" plane through (27, 12, -39.875) normal (0, 1, 0) x (1, 0, 0)
  line L0 (-21.75, 0) -> (-22.75, 0)
  line L1 (-22.75, 0) -> (-22.75, 9.875)
  line L2 (-22.75, 9.875) -> (-21.75, 9.875)
  line L3 (-21.75, 9.875) -> (-21.75, 0)
  line L4 (-32.25, 0) -> (-31.25, 0)
  line L5 (-31.25, 0) -> (-31.25, 9.875)
  line L6 (-31.25, 9.875) -> (-32.25, 9.875)
  line L7 (-32.25, 9.875) -> (-32.25, 0)
  line L8 (-21.75, 9.875) -> (-32.25, 9.875) projected
  line L9 (-32.25, 0) -> (-21.75, 0) projected
  line L10 (-21.75, 0) -> (-21.75, 9.875) projected
  line L11 (-32.25, 9.875) -> (-32.25, 0) projected
  point P0 (-27, -39.875)
  dimension "d331" = 1
  constraints: 16 end point, 7 collinear, 4 parallel, 2 horizontal, 2 perpendicular
  measures "d331" distance of L5.end L6.end
extrude "Vysunutí56" add sketch "Náčrt54" along normal blind 1 contours L0 L1 L2 L3 | L4 L7 L6 L5
chamfer "Zkosení10" distance 1 angle 45 1 edges at (-1.85, 10, -44.8125)
sketch "Náčrt56" plane through (0, 0, 0) normal (0, -1, 0) x (1, 0, 0)
  line L0 (27, -19.25) -> (27, -39.75) projected
  line L1 (49.75, -19.25) -> (27, -19.25) projected
  line L2 (49.75, 49.75) -> (49.75, -19.25) projected
  line L3 (-49.75, 49.75) -> (49.75, 49.75) projected
  line L4 (-49.75, -19.25) -> (-49.75, 49.75) projected
  line L5 (-27, -19.25) -> (-49.75, -19.25) projected
  line L6 (-27, -39.75) -> (-27, -19.25) projected
  line L7 (27, -39.75) -> (27, -46.75) projected
  line L8 (-27, -46.75) -> (-27, -39.75) projected
  line L9 (-27, -49.75) -> (-27, -46.75) projected
  line L10 (27, -46.75) -> (27, -49.75) projected
  line L11 (27, -49.75) -> (-27, -49.75) projected
  line L12 (-27, -49.75) -> (-27, -39.875) projected
  line L13 (-27, -39.75) -> (27, -39.75) projected
extrude "Vysunutí57" cut sketch "Náčrt56" against normal blind 3 contours L0 L13 L6 L5 L4 L3 L2 L1 keep common part
chamfer "Zkosení12" distance 0.5 angle 45 16 edges at (49.75, 0, 15.25) (49.75, 3, 14.8481) (27, 0, -29.5) (38.375, 0, -19.25) (38.375, 3, -19.25) (27, 3, -29.5) (0, 3, -39.75) (0, 0, -39.75) (-27, 3, -29.5) (-38.375, 3, -19.25) (-38.375, 0, -19.25) (-27, 0, -29.5) (-49.75, 0, 15.25) (-49.75, 3, 14.8481) (0, 3, 48.9462) (0, 0, 49.75)
